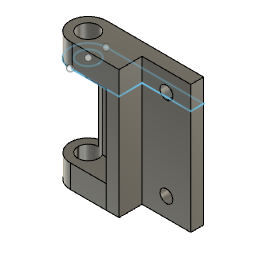
hinge2 v2 (Autodesk Fusion 360 design; units mm, degrees)
Autodesk Fusion 360 part; units mm, degrees
sketch "Sketch1" plane through (0, 0, 0) normal (0, 0, 1) x (1, 0, 0)
  line L0 (-25, -3) -> (13, -3)
  circle A0 centre (-25, 11) radius 8
  line L1 (-25, 25.2064) -> (-25, 24.9277)
  line L2 (-25, -2.9277) -> (-25, -3)
  arc A1 (-25, 25.0771) -> (-23.5283, -3) centre (-25, 11) ccw
  line L3 (13, -3) -> (13, 15)
  line L4 (13, 15) -> (51, 15)
  line L5 (51, 15) -> (51, 25)
  line L6 (51, 25) -> (-25, 25.2064)
  dimension "d12" = 18
  dimension "d33" = 10
  constraint concentric A0 A1
  constraint coincident L0 A1.end
  constraint coincident L1 A1.start
  constraint perpendicular L0 L3
  constraint perpendicular L4 L5
  measures "d12" distance of L0.end L3.end
  measures "d33" distance of L4.end L5.end
extrude "Extrude7" add sketch "Sketch1" along normal blind 18
sketch "Sketch8" plane through (51, 0, 0) normal (1, 0, 0) x (0, 1, 0)
  line L0 (15, 0) -> (25, 0)
  line L1 (25, 0) -> (25, 18)
  line L2 (25, 18) -> (15, 18)
  line L3 (15, 18) -> (15, 0)
  line L4 (25, 0) -> (25, -82)
  line L5 (15, 0) -> (15, -82)
  line L6 (25, -82) -> (15, -82)
  constraint coincident L0.end L1.start
  constraint perpendicular L0 L4
  constraint coincident L0.start L3.end
  constraint perpendicular L0 L5
  constraint perpendicular L5 L6
extrude "Extrude8" add sketch "Sketch8" against normal blind 76 contours L0 L4 L5 L6
sketch "Sketch9" plane through (13, 0, 0) normal (1, 0, 0) x (0, 1, 0)
  line L0 (-3, 0) -> (15, 0)
  line L1 (15, 0) -> (15, 18)
  line L2 (15, 18) -> (-3, 18)
  line L3 (-3, 18) -> (-3, 0)
  line L4 (-3, 0) -> (-3, -82)
  line L5 (15, 0) -> (15, -82)
  line L6 (-3, -82) -> (15, -82)
  constraint coincident L0.start L3.end
  constraint perpendicular L0 L4
  constraint coincident L0.end L1.start
  constraint perpendicular L0 L5
  constraint perpendicular L5 L6
sketch "Sketch13" plane through (13, 0, 0) normal (1, 0, 0) x (0, 1, 0)
  line L0 (-3, 0) -> (15, 0)
  line L1 (15, 0) -> (15, 18)
  line L2 (15, 18) -> (-3, 18)
  line L3 (-3, 18) -> (-3, 0)
  line L4 (-3, 0) -> (-3, -82)
  line L5 (15, 0) -> (15, -82)
  line L6 (-3, -82) -> (15, -82)
  constraint coincident L0.start L3.end
  constraint perpendicular L0 L4
  constraint coincident L0.end L1.start
  constraint perpendicular L0 L5
  constraint perpendicular L5 L6
extrude "Extrude12" add sketch "Sketch13" against normal blind 10 contours L0 L4 L5 L6
sketch "Sketch14" plane through (0, 0, -82) normal (0, 0, -1) x (1, 0, 0)
  line L0 (51, -25) -> (51, -15)
  line L1 (51, -15) -> (13, -15)
  line L2 (13, -15) -> (13, 3)
  line L3 (13, 3) -> (3, 3)
  line L4 (3, 3) -> (3, -15)
  line L5 (3, -15) -> (-25, -15)
  line L6 (-25, -15) -> (-25, -25)
  line L7 (-25, -25) -> (51, -25)
  line L8 (3, -15) -> (-25, -15)
  line L9 (-25, -15) -> (3, -15)
  line L10 (3, 3) -> (3, -15)
  line L11 (-25, 3) -> (3, 3)
  circle A0 centre (-25, -10.9541) radius 8
  arc A1 (-24.761, 3) -> (-25, -24.9103) centre (-25, -10.9541) ccw
  dimension "d54" = 16
  constraint coincident L4.end L5.start
  constraint coincident L5.end L6.start
  constraint coincident L3.end L4.start
  constraint concentric A0 A1
  constraint coincident L11 A1.start
  constraint coincident L6 A1.end
  measures "d54" diameter of A0
extrude "Extrude13" add sketch "Sketch14" against normal blind 18 contours L4 L5 L6 L8 L9 L10 L11 A0 A1
hole "Hole1" at (-25, 10.9541, -82) direction (0, 0, 1) diameter 16 depth 18 tip angle 118
hole "Hole2" at (-25, 11, 18) direction (0, 0, -1) diameter 16 depth 100 tip angle 118
sketch "Sketch15" plane through (0, 15, 0) normal (0, -1, 0) x (1, 0, 0)
  line L0 (13, 18) -> (13, -82)
  line L1 (13, -82) -> (51, -82)
  line L2 (51, -82) -> (51, 18)
  line L3 (51, 18) -> (13, 18)
  line L4 (32, 8) -> (32, 3)
  line L5 (32, -72) -> (32, -67)
  circle A0 centre (32, 3) radius 5
  circle A1 centre (32, -67) radius 5
  dimension "d66" = 10
  constraint perpendicular L3 L4
  constraint perpendicular L1 L5
  constraint coincident L4.end A0.centre
  constraint coincident L5.end A1.centre
  constraint coincident A0 L4.start
  constraint coincident A1 L5.start
  measures "d66" diameter of A1
extrude "Extrude14" cut sketch "Sketch15" against normal blind 10 contours A0
hole "Hole3" at (32.0476, 25.0515, 3.0029) direction (-0.002716, -0.999996, 0) diameter 10 depth 10 tip angle 118
sketch "Sketch16" plane through (0, 15, 0) normal (0, -1, 0) x (1, 0, 0)
  circle A0 centre (32, 3) radius 5
  line L0 (13, 18) -> (13, -82)
  line L1 (13, -82) -> (51, -82)
  line L2 (51, -82) -> (51, 18)
  line L3 (51, 18) -> (13, 18)
  circle A1 centre (32, -67) radius 5
extrude "Extrude15" cut sketch "Sketch16" against normal blind 10 contours A1
extrude "Extrude9" [suppressed]
sketch "Sketch10" plane through (-25, 0, 0) normal (-1, 0, 0) x (0, -1, 0)
  line L0 (-3, 0) -> (-19, 0)
  line L1 (-19, 0) -> (-25, 0)
  line L2 (-25, 0) -> (-25, -82)
  line L3 (-25, -82) -> (3, -82)
  line L4 (3, -82) -> (3, 0)
  line L5 (3, 0) -> (-3, 0)
sketch "Sketch11" plane through (0, 0, -82) normal (0, 0, -1) x (1, 0, 0)
  line L0 (51, -25) -> (51, -15)
  line L1 (51, -15) -> (13, -15)
  line L2 (13, -15) -> (13, 3)
  line L3 (13, 3) -> (-25, 3)
  line L4 (-25, 3) -> (-25, -25)
  line L5 (-25, -25) -> (51, -25)
  circle A0 centre (-25, -11) radius 8
  arc A1 (-25, 2.9906) -> (-25, -24.9906) centre (-25, -11) ccw
  constraint midpoint L4 A0.centre
  constraint concentric A0 A1
  constraint coincident L4 A1.end
  constraint coincident L4 A1.start
extrude "Extrude10" [suppressed]
sketch "Sketch12" plane through (0, 0, -82) normal (0, 0, -1) x (1, 0, 0)
  line L0 (51, -25) -> (51, -15)
  line L1 (51, -15) -> (13, -15)
  line L2 (13, -15) -> (13, 3)
  line L3 (13, 3) -> (-25, 3)
  line L4 (-25, 3) -> (-25, -25)
  line L5 (-25, -25) -> (51, -25)
  arc A0 (-25, 2.9695) -> (-25, -24.9695) centre (-25, -11) ccw
  constraint midpoint L4 A0.centre
  constraint coincident L4 A0.end
  constraint coincident L4 A0.start
extrude "Extrude11" [suppressed]
extrude "Extrude1" [suppressed]
sketch "Sketch2" plane through (51, 0, 0) normal (1, 0, 0) x (0, 1, 0)
  line L0 (15, 0) -> (25.2064, 0)
  line L1 (25.2064, 0) -> (25.2064, 18)
  line L2 (25.2064, 18) -> (15, 18)
  line L3 (15, 18) -> (15, 0)
  line L4 (15, 0) -> (15, -82)
  line L5 (25.2064, 0) -> (25.2064, -82)
  line L6 (15, -82) -> (25.2064, -82)
  constraint coincident L0.start L3.end
  constraint perpendicular L0 L4
  constraint coincident L0.end L1.start
  constraint perpendicular L0 L5
sketch "Sketch3" plane through (13, 0, 0) normal (1, 0, 0) x (0, 1, 0)
  line L0 (-3, 0) -> (15, 0)
  line L1 (15, 0) -> (15, 18)
  line L2 (15, 18) -> (-3, 18)
  line L3 (-3, 18) -> (-3, 0)
  line L4 (15, 0) -> (15, -82)
  line L5 (-3, 0) -> (-3, -82)
  line L6 (15, -82) -> (-3, -82)
  constraint coincident L0.end L1.start
  constraint perpendicular L0 L4
  constraint coincident L0.start L3.end
  constraint perpendicular L0 L5
  constraint perpendicular L5 L6
extrude "Extrude2" [suppressed]
sketch "Sketch4" plane through (51, 0, 0) normal (1, 0, 0) x (0, 1, 0)
extrude "Extrude3" [suppressed]
other "Form1"
sketch "Sketch5" plane through (0, 0, 0) normal (1, 0, 0) x (0, 1, 0)
extrude "Extrude4" [suppressed]
sketch "Sketch6" plane through (0, 25.2064, 0) normal (0, 1, 0) x (-1, 0, 0)
  line L0 (19, 0) -> (25, 0)
  line L1 (25, 0) -> (25, 18)
  line L2 (25, 18) -> (-51, 18)
  line L3 (-51, 18) -> (-51, -82)
  line L4 (-51, -82) -> (19, -82)
  line L5 (19, -82) -> (19, 0)
  line L6 (25, 0) -> (25, -82)
  line L7 (19, 0) -> (19, -82)
  line L8 (19, -82) -> (25, -82)
  dimension "d26" = 82
  dimension "d27" = 82
  constraint coincident L0.end L1.start
  constraint perpendicular L0 L6
  constraint coincident L0.start L5.end
  constraint perpendicular L0 L7
  measures "d26" distance of L0.end L6.end
  measures "d27" distance of L0.start L4.end
extrude "Extrude5" [suppressed]
extrude "Extrude6" [suppressed]
sketch "Sketch7" plane through (-23.258, 0, 0) normal (-1, 0, 0) x (0, -1, 0)
  line L0 (3, -82) -> (3, 0)
  line L1 (3, 0) -> (-3.192, 0)
  line L2 (-3.192, 0) -> (-15, 0)
  line L3 (-15, 0) -> (-15, -82)
  line L4 (-15, -82) -> (3, -82)
